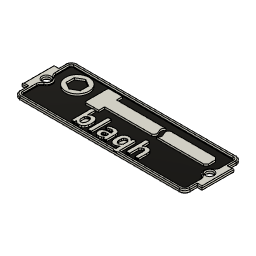
gridfinity_label_parametric_legacy (Autodesk Fusion 360 design; units mm, degrees)
Autodesk Fusion 360 part; units mm, degrees
sketch "Sketch1" plane through (0, 0, 35.65) normal (0, 0, 1) x (-1, 0, 0)
  line L0 (-2.15, 2.65) -> (-18.9, 2.65)
  line L1 (-0.25, -3.35) -> (-0.25, -0.5)
  line L2 (-1.25, -0.5) -> (-1.25, 1.5)
  arc A0 (-1.25, 1.5) -> (-2.15, 2.4) centre (-2.15, 1.5) ccw
  line L3 (-2.15, 2.4) -> (-18.9, 2.4)
  line L4 (-1.25, -0.5) -> (-0.25, -0.5)
  line L5 (0, -3.35) -> (0, 0)
  line L6 (0, 0) -> (-1, 0)
  line L7 (-1, 0) -> (-1, 1.5)
  arc A1 (-1, 1.5) -> (-2.15, 2.65) centre (-2.15, 1.5) ccw
  line L8 (-18.9, -3.35) -> (-18.9, 2.65)
  line L9 (0, -3.35) -> (-18.9, -3.35)
  line L10 (0, 0) -> (-24, 0) construction
  line L11 (0, -3.35) -> (0, -6.7)
  line L12 (-1, -6.7) -> (-1, -8.2)
  line L13 (0, -3.35) -> (-18.9, -3.35)
  line L14 (-1.25, -6.2) -> (-0.25, -6.2)
  arc A2 (-2.15, -9.35) -> (-1, -8.2) centre (-2.15, -8.2) ccw
  line L15 (-2.15, -9.35) -> (-18.9, -9.35)
  line L16 (-1.25, -6.2) -> (-1.25, -8.2)
  line L17 (0, -6.7) -> (-1, -6.7)
  arc A3 (-2.15, -9.1) -> (-1.25, -8.2) centre (-2.15, -8.2) ccw
  line L18 (-0.25, -3.35) -> (-0.25, -6.2)
  line L19 (-2.15, -9.1) -> (-18.9, -9.1)
  line L20 (-18.9, -3.35) -> (-18.9, -9.35)
  line L21 (-36.55, -6.2) -> (-37.55, -6.2)
  line L22 (-37.8, -6.7) -> (-36.8, -6.7)
  line L23 (-35.65, -9.35) -> (-18.9, -9.35)
  line L24 (-37.8, -3.35) -> (-18.9, -3.35)
  line L25 (-36.8, 0) -> (-36.8, 1.5)
  line L26 (-35.65, 2.4) -> (-18.9, 2.4)
  line L27 (-36.55, -0.5) -> (-37.55, -0.5)
  line L28 (-35.65, 2.65) -> (-18.9, 2.65)
  arc A4 (-35.65, 2.4) -> (-36.55, 1.5) centre (-35.65, 1.5) ccw
  line L29 (-37.55, -3.35) -> (-37.55, -6.2)
  line L30 (-37.55, -3.35) -> (-37.55, -0.5)
  line L31 (-37.8, -3.35) -> (-18.9, -3.35)
  line L32 (-36.55, -6.2) -> (-36.55, -8.2)
  arc A5 (-36.55, -8.2) -> (-35.65, -9.1) centre (-35.65, -8.2) ccw
  line L33 (-37.8, -3.35) -> (-37.8, 0)
  line L34 (-18.9, -3.35) -> (-18.9, 2.65)
  line L35 (-37.8, 0) -> (-36.8, 0)
  arc A6 (-35.65, 2.65) -> (-36.8, 1.5) centre (-35.65, 1.5) ccw
  arc A7 (-36.8, -8.2) -> (-35.65, -9.35) centre (-35.65, -8.2) ccw
  line L36 (-36.55, -0.5) -> (-36.55, 1.5)
  line L37 (-35.65, -9.1) -> (-18.9, -9.1)
  line L38 (-36.8, -6.7) -> (-36.8, -8.2)
  line L39 (-18.9, -3.35) -> (-18.9, -9.35)
  line L40 (-37.8, -3.35) -> (-37.8, -6.7)
  point P0 (0, -6.7)
  point P1 (0, -6.7)
  point P2 (-37.8, -6.7)
  point P3 (-37.8, -6.7)
  point P4 (-37.8, 0)
  point P5 (-37.8, 0)
  dimension "d562" = 0.25
  dimension "d566" = 0.5
  dimension "d4" = 18.9
  dimension "d5" = 3.35
  dimension "d6" = 1
  dimension "d7" = 1
  dimension "d8" = 1.15
  dimension "d9" = 0.9
  dimension "d10" = 2
  dimension "d11" = 1.5
  dimension "d12" = 0.9
  dimension "d13" = 1.15
  constraint coincident L1 L4.end
  constraint perpendicular L1 L4
  constraint tangent L2 A0
  constraint tangent A0 L3
  constraint coincident A0.centre A1.centre
  constraint coincident L5.end L6.start
  constraint coincident L8 L3.end
  constraint coincident L9 L1.start
  constraint parallel L0 L3
  constraint perpendicular L6 L7
  constraint perpendicular L5 L9
  constraint parallel L9 L10
  constraint symmetric L5.end L9 P1
  constraint symmetric L0.start L9 A2.start
  constraint symmetric L2.end L9 L16.end
  constraint symmetric A0.end L9 A3.start
  constraint symmetric A0 L9 A3
  constraint symmetric L2.start L9 L14.start
  constraint symmetric L1.end L9 L14.end
  constraint symmetric L6.end L9 L12.start
  constraint symmetric L7.end L9 L12.end
  constraint symmetric A1 L9 A2
  constraint symmetric L5.start L9 L11.start
  constraint symmetric L8.start L9 L13.end
  constraint symmetric L0.end L9 L15.end
  constraint symmetric L3.end L9 L19.end
  constraint symmetric L9 L1.start L18.start
  constraint symmetric L9 L5.end P1
  constraint symmetric L5.end L20 P5
  constraint symmetric L0.start L20 L28.start
  constraint symmetric L2.end L20 A4.end
  constraint symmetric A0.end L20 L26.start
  constraint symmetric A0 L20 A4
  constraint symmetric L2.start L20 L27.start
  constraint symmetric L1.end L20 L27.end
  constraint symmetric L6.end L20 L25.start
  constraint symmetric L7.end L20 L25.end
  constraint symmetric A1 L20 A6
  constraint symmetric L5.start L20 L24.start
  constraint symmetric L8.start L20 L9.end
  constraint symmetric L0.end L20 L8.end
  constraint symmetric L3.end L20 L26.end
  constraint symmetric L1.start L20 L29.start
  constraint symmetric L15.end L20 L23.end
  constraint symmetric A3.start L20 A5.end
  constraint symmetric L12.end L20 A7.start
  constraint symmetric P1 L20 P3
  constraint symmetric L12.start L20 L22.end
  constraint symmetric L19.end L20 L37.end
  constraint symmetric L16.end L20 L32.end
  constraint symmetric L14.end L20 L21.end
  constraint symmetric A2.start L20 L23.start
  constraint symmetric L14.start L20 L21.start
  constraint symmetric A2 L20 A7
  constraint symmetric A3 L20 A5
  constraint perpendicular L3 L34
  measures "d562" distance of L1 L5
  measures "d566" distance of L4 L6
  measures "d4" distance of L5.start L8.start
  measures "d5" distance of L5.end L5.start
  measures "d6" distance of L5.end L6.end
  measures "d7" distance of L2.start L1.end
  measures "d8" radius of A1
  measures "d9" radius of A0
  measures "d10" distance of L2.end L2.start
  measures "d11" distance of L6.end L7.end
  measures "d12" distance of L2 A0.end
  measures "d13" horizontal distance of L0.start L7.end
extrude "Extrude1" add sketch "Sketch1" along normal blind 0.4 makes body 1
sketch "Sketch2" plane through (0, 0, 36.05) normal (0, 0, 1) x (-1, 0, 0)
  line L0 (-2.15, -8.6) -> (-35.65, -8.6)
  line L1 (-36.05, -8.2) -> (-36.05, 1.5)
  line L2 (-35.65, 1.9) -> (-2.15, 1.9)
  line L3 (-1.75, 1.5) -> (-1.75, -8.2)
  arc A0 (-2.15, -8.6) -> (-1.75, -8.2) centre (-2.15, -8.2) ccw
  arc A1 (-1.75, 1.5) -> (-2.15, 1.9) centre (-2.15, 1.5) ccw
  arc A2 (-35.65, 1.9) -> (-36.05, 1.5) centre (-35.65, 1.5) ccw
  arc A3 (-36.05, -8.2) -> (-35.65, -8.6) centre (-35.65, -8.2) ccw
  circle A4 centre (-1.75, -3.35) radius 0.75
  circle A5 centre (-36.05, -3.35) radius 0.75
  circle A6 centre (-1.75, -3.35) radius 1.25
  circle A7 centre (-36.05, -3.35) radius 1.25
  arc A8 (-2.15, -9.35) -> (-1, -8.2) centre (-2.15, -8.2) ccw
  line L4 (-1, -8.2) -> (-1, -6.7)
  line L5 (-1, -6.7) -> (0, -6.7)
  line L6 (0, -6.7) -> (0, 0)
  line L7 (0, 0) -> (-1, 0)
  line L8 (-1, 0) -> (-1, 1.5)
  arc A9 (-1, 1.5) -> (-2.15, 2.65) centre (-2.15, 1.5) ccw
  arc A10 (-35.65, 2.65) -> (-36.8, 1.5) centre (-35.65, 1.5) ccw
  line L9 (-2.15, 2.65) -> (-35.65, 2.65)
  arc A11 (-35.65, 2.65) -> (-36.8, 1.5) centre (-35.65, 1.5) ccw
  line L10 (-36.8, 1.5) -> (-36.8, 0)
  line L11 (-36.8, 0) -> (-37.8, 0)
  line L12 (-37.8, 0) -> (-37.8, -6.7)
  line L13 (-37.8, -6.7) -> (-36.8, -6.7)
  line L14 (-36.8, -6.7) -> (-36.8, -8.2)
  arc A12 (-36.8, -8.2) -> (-35.65, -9.35) centre (-35.65, -8.2) ccw
  line L15 (-35.65, -9.35) -> (-2.15, -9.35)
  point P0 (-2.15, -8.2)
  dimension "d517" = 1.5
  dimension "d518" = 2.5
  constraint horizontal L0
  constraint vertical L1
  constraint horizontal L2
  constraint vertical L3
  constraint tangent L0 A0
  constraint tangent L3 A0
  constraint tangent L3 A1
  constraint tangent L2 A1
  constraint equal A0 A1
  constraint tangent L2 A2
  constraint tangent L1 A2
  constraint equal A0 A2
  constraint tangent L1 A3
  constraint tangent L0 A3
  constraint equal A0 A3
  constraint midpoint L3 A4.centre
  constraint midpoint L1 A5.centre
  constraint concentric A4 A6
  constraint concentric A5 A7
  constraint equal A4 A5
  constraint equal A6 A7
  constraint coincident P0 A0.centre
  constraint concentric A2 A10
  measures "d517" diameter of A4
  measures "d518" diameter of A6
extrude "Extrude2" add sketch "Sketch2" along normal blind 0.4 contours L3 A4 A6 | L3 A4 A6 | L1 A5 A7 | L1 A5 A7 | L3 A4 | L3 A4 | L1 A5 | L1 A5 | A8 L4 L5 L6 L7 L8 A9 A10 L9 A11 L10 L11 L12 L13 L14 A12 L15 bodies 1
fillet "Fillet2" radius 1 4 edges at (1.75, 2.1, 36.25) (1.75, 4.6, 36.25) (36.05, 2.1, 36.25) (36.05, 4.6, 36.25) on bodies 1
extrude "Extrude4" cut sketch "Sketch2" along normal through all and the other way through all contours L3 A4 | L3 A4 | L1 A5 | L1 A5 bodies 1
fillet "Fillet1" radius 0.2 2 faces at (37.4667, 3.35, 36.45) (13.4333, 3.35, 35.65) on bodies 1
sketch "Sketch3" plane through (0, 0, 36.05) normal (0, 0, 1) x (-1, 0, 0)
  line L0 (-35.65, -8.6) -> (-2.15, -8.6)
  line L1 (-2.15, 1.9) -> (-35.65, 1.9)
  line L2 (-2.15, -8.6) -> (-35.65, -8.6) construction
  line L3 (-35.65, -8.6) -> (-35.65, 1.9) construction
  line L4 (-35.65, 1.9) -> (-2.15, 1.9) construction
  line L5 (-2.15, 1.9) -> (-2.15, -8.6) construction
  line L6 (-2.15, -3.35) -> (-35.65, -3.35) construction
  arc A0 (-35.4944, -4.4698) -> (-36.05, -5.3656) centre (-35.05, -5.3656) ccw
  line L7 (-36.05, -5.3656) -> (-36.05, -8.2)
  arc A1 (-36.05, -8.2) -> (-35.65, -8.6) centre (-35.65, -8.2) ccw
  arc A2 (-2.15, -8.6) -> (-1.75, -8.2) centre (-2.15, -8.2) ccw
  line L8 (-1.75, -8.2) -> (-1.75, -5.3656)
  arc A3 (-1.75, -5.3656) -> (-2.3056, -4.4698) centre (-2.75, -5.3656) ccw
  arc A4 (-2.3056, -2.2302) -> (-2.3056, -4.4698) centre (-1.75, -3.35) ccw
  arc A5 (-2.3056, -2.2302) -> (-1.75, -1.3344) centre (-2.75, -1.3344) ccw
  line L9 (-1.75, -1.3344) -> (-1.75, 1.5)
  arc A6 (-1.75, 1.5) -> (-2.15, 1.9) centre (-2.15, 1.5) ccw
  arc A7 (-35.65, 1.9) -> (-36.05, 1.5) centre (-35.65, 1.5) ccw
  line L10 (-36.05, 1.5) -> (-36.05, -1.3344)
  arc A8 (-36.05, -1.3344) -> (-35.4944, -2.2302) centre (-35.05, -1.3344) ccw
  arc A9 (-35.4944, -4.4698) -> (-35.4944, -2.2302) centre (-36.05, -3.35) ccw
  line L11 (-2.15, -5.6) -> (-35.65, -5.6) construction
  line L12 (-18.9, -8.6) -> (-18.9, -5.6) construction
  line L13 (-18.9, -5.6) -> (-18.9, -3.35) construction
  line L14 (-34.3, -5.6) -> (-13, -5.6)
  line L15 (-13, -5.6) -> (-13, -6.85)
  line L16 (-13, -6.85) -> (-33.8, -6.85)
  line L17 (-34.3, -6.35) -> (-34.3, -5.6)
  line L18 (-13, -5.6) -> (-10, -5.6)
  line L19 (-10, -5.6) -> (-10, -7.8)
  line L20 (-10.3, -8.1) -> (-13, -8.1)
  line L21 (-13, -8.1) -> (-13, -5.6)
  circle A10 centre (-6, -5.6) radius 2.5
  line L22 (-7.5, -6.466) -> (-6, -7.3321)
  line L23 (-6, -7.3321) -> (-4.5, -6.466)
  line L24 (-4.5, -6.466) -> (-4.5, -4.734)
  line L25 (-4.5, -4.734) -> (-6, -3.8679)
  line L26 (-6, -3.8679) -> (-7.5, -4.734)
  line L27 (-7.5, -4.734) -> (-7.5, -6.466)
  arc A11 (-10.3, -8.1) -> (-10, -7.8) centre (-10.3, -7.8) ccw
  line L28 (-2.15, 1.5) -> (-35.65, 1.5) construction
  line L29 (-35.65, 1.5) -> (-35.65, -3.35) construction
  line L30 (-35.65, -3.35) -> (-2.15, -3.35) construction
  line L31 (-2.15, -3.35) -> (-2.15, 1.5) construction
  line L32 (-33.8, -6.85) -> (-34.3, -6.35)
  line L33 (-10, -5.6) -> (-10, -3.4)
  line L34 (-13, -3.1) -> (-13, -5.6)
  line L35 (-18.9, -2.6) -> (-18.9, -5.6) construction
  line L36 (-13, -4.35) -> (-33.8, -4.35)
  line L37 (-34.3, -4.85) -> (-34.3, -5.6)
  line L38 (-13, -5.6) -> (-10, -5.6)
  line L39 (-10.3, -3.1) -> (-13, -3.1)
  line L40 (-13, -5.6) -> (-13, -4.35)
  line L41 (-34.3, -5.6) -> (-13, -5.6)
  arc A12 (-10, -3.4) -> (-10.3, -3.1) centre (-10.3, -3.4) ccw
  line L42 (-33.8, -4.35) -> (-34.3, -4.85)
  point P0 (-34.3, -6.85)
  point P1 (-10, -8.1)
  point P2 (-6, -5.6)
  point P3 (-10, -3.1)
  point P4 (-34.3, -4.35)
  dimension "d21" = 3
  dimension "d22" = 0.4
  dimension "d23" = 21.3
  dimension "d24" = 3
  dimension "d25" = 1.25
  dimension "d26" = 2.5
  dimension "d31" = 5
  dimension "d33" = 1.5
  dimension "d34" = 4
  dimension "d38" = 33.5
  dimension "d39" = 1.35
  dimension "d41" = 0.3
  dimension "d43" = 4
  dimension "d44" = 0.4
  dimension "d45" = 0.5
  dimension "d46" = 0.5
  dimension "d67" = 0.4
  text T0 "blaqh" font "Calibri" height 4 bold align centre bottom in box 33.5 x 4.85 at (-2.15, 1.5) x (-1, 0) y (0, -1) spacing 1 kerned
  constraint horizontal L2
  constraint vertical L3
  constraint horizontal L4
  constraint vertical L5
  constraint midpoint L5 L6.start
  constraint midpoint L3 L6.end
  constraint coincident L5 L11.start
  constraint coincident L3 L11.end
  constraint perpendicular L3 L11
  constraint midpoint L2 L12.start
  constraint midpoint L11 L12.end
  constraint horizontal L14
  constraint vertical L15
  constraint horizontal L16
  constraint vertical L17
  constraint coincident L11 L14.start
  constraint horizontal L18
  constraint vertical L19
  constraint horizontal L20
  constraint vertical L21
  constraint coincident L11 P2
  constraint coincident P2 A10.centre
  constraint coincident P1 L19
  constraint coincident P1 L20
  constraint tangent L19 A11
  constraint tangent L20 A11
  constraint coincident L1.start L4
  constraint coincident L5
  constraint coincident L6.end
  constraint coincident P0 L16
  constraint coincident P0 L17
  constraint symmetric L11 L12.start L35.start
  constraint symmetric L11 L12.end L13.start
  constraint symmetric L11 L14.start L17.end
  constraint symmetric L11 L14.end L15.start
  constraint symmetric L11 L15.end L36.start
  constraint symmetric L11 P0 P4
  constraint symmetric L11 L18.end L19.start
  constraint symmetric L11 P1 P3
  constraint symmetric L11 L20.end L34.start
  constraint symmetric L11 L19.end L33.end
  constraint symmetric L11 L20.start L39.start
  constraint symmetric L11 A11 A12
  constraint symmetric L11 L16.end L36.end
  constraint symmetric L11 L17.start L37.start
  measures "d21" distance of L0 L11
  measures "d22" distance of L8 L11.start
  measures "d23" distance of L15.end P0
  measures "d24" distance of P1 L20.end
  measures "d25" distance of L14 L16
  measures "d26" distance of L18.end P1
  measures "d31" diameter of A10
  measures "d33" distance of P2 L27
  measures "d34" distance of L19 P2
  measures "d38" distance of L0.end L0.start
  measures "d39" distance of L3 L17
  measures "d41" radius of A11
  measures "d44" distance of L4 L28
  measures "d45" distance of P0 L16.end
  measures "d46" distance of P0 L17.start
  measures "d67" distance of L3 L7
extrude "Extrude3" add sketch "Sketch3" sketch "Sketch3" along normal blind 0.4 contours L14 L34 L36 L37 L40 L41 L42 | L14 L15 L16 L17 L21 L32 L41 | L15 L18 L19 L20 L21 A11 L38 | L18 L33 L34 L38 L39 L40 A12 | A10 of sketch 2 text T0 bodies 1
sketch "Skizze4" plane through (0, 0, 36.45) normal (0, 0, 1) x (-1, 0, 0)
  line L0 (-12.988, -6.85) -> (-12.988, -5.6) construction
  line L1 (-12.988, -5.6) -> (-34.3, -5.6) construction
  spline S0 degree 5 poles (-23.398, -6.85) (-23.3526, -6.8257) (-23.2673, -6.7758) (-23.156, -6.6971) (-23.0412, -6.5844) (-22.9541, -6.4303) (-22.9227, -6.2632) (-22.9431, -6.0841) (-23.0069, -5.8949) (-23.099, -5.6991) (-23.201, -5.5009) (-23.2931, -5.3051) (-23.3569, -5.1159) (-23.3773, -4.9368) (-23.3459, -4.7697) (-23.2588, -4.6156) (-23.144, -4.5029) (-23.0327, -4.4242) (-22.9474, -4.3743) (-22.902, -4.35) knots 0 0 0 0 0 0 0.066667 0.133333 0.2 0.266667 0.333333 0.4 0.466667 0.533333 0.6 0.666667 0.733333 0.8 0.866667 0.933333 1 1 1 1 1 1
  spline S1 degree 5 poles (-24.398, -6.85) (-24.3526, -6.8257) (-24.2673, -6.7758) (-24.156, -6.6971) (-24.0412, -6.5844) (-23.9541, -6.4303) (-23.9227, -6.2632) (-23.9431, -6.0841) (-24.0069, -5.8949) (-24.099, -5.6991) (-24.201, -5.5009) (-24.2931, -5.3051) (-24.3569, -5.1159) (-24.3773, -4.9368) (-24.3459, -4.7697) (-24.2588, -4.6156) (-24.144, -4.5029) (-24.0327, -4.4242) (-23.9474, -4.3743) (-23.902, -4.35) knots 0 0 0 0 0 0 0.066667 0.133333 0.2 0.266667 0.333333 0.4 0.466667 0.533333 0.6 0.666667 0.733333 0.8 0.866667 0.933333 1 1 1 1 1 1
  line L2 (-23.65, -5.6) -> (-22.95, -6.1)
  line L3 (-23.65, -5.6) -> (-23.95, -6.1)
  line L4 (-24.35, -5.1) -> (-23.65, -5.6)
  line L5 (-23.35, -5.1) -> (-23.65, -5.6)
  line L6 (-12.988, -5.6) -> (-12.988, -4.35) construction
  line L7 (-10, -7.8) -> (-10, -3.4)
  arc A0 (-10, -3.4) -> (-10.3, -3.1) centre (-10.3, -3.4) ccw
  line L8 (-10.3, -3.1) -> (-13, -3.1)
  line L9 (-13, -3.1) -> (-13, -4.35)
  line L10 (-13, -4.35) -> (-33.8, -4.35)
  line L11 (-33.8, -4.35) -> (-34.3, -4.85)
  line L12 (-34.3, -4.85) -> (-34.3, -6.35)
  line L13 (-34.3, -6.35) -> (-33.8, -6.85)
  line L14 (-33.8, -6.85) -> (-13, -6.85)
  line L15 (-13, -6.85) -> (-13, -8.1)
  line L16 (-13, -8.1) -> (-10.3, -8.1)
  arc A1 (-10.3, -8.1) -> (-10, -7.8) centre (-10.3, -7.8) ccw
  line L17 (-23.398, -6.85) -> (-24.398, -6.85)
  line L18 (-22.902, -4.35) -> (-23.902, -4.35)
  point P0 (-22.95, -6.1)
  point P1 (-23.35, -5.1)
  point P2 (-29.15, -5.6164)
  point P3 (-23.95, -6.1)
  point P4 (-24.35, -5.1)
  dimension "d48" = 0.5
  dimension "d49" = 0.5
  dimension "d50" = 0.448
  dimension "d51" = 0.448
  dimension "d52" = 0.4
  dimension "d56" = -1
  dimension "d57" = 0
  dimension "d70" = 10.65
  constraint coincident P4 L4.start
  constraint coincident P0 L2.end
  constraint coincident P1 L5.start
  constraint coincident P3 L3.end
  constraint equal L2 L4
  constraint equal L3 L5
  constraint equal L0 L6
  constraint perpendicular L1 L6
  constraint coincident S0.start L14
  constraint coincident S0.end L10
  constraint coincident L0.start L14
  constraint coincident L6.end L10
  constraint parallel L1 L14
  constraint parallel L0 L6
  measures "d48" distance of L1 P0
  measures "d49" distance of L1 P1
  measures "d50" distance of S0.start P0
  measures "d51" distance of P1 S0.end
  measures "d52" horizontal distance of P0 P1
  measures "d70" distance of L2.start L12
extrude "Extrusion5" add sketch "Skizze4" along normal blind 0.4 separate body contours S0 S1 L2 L3 L14 L17 | S0 L2 L5 | S0 S1 L4 L5 L10 L18 | S1 L3 L4 makes body 2
move_body "Verschieben1" bodies 2 to x (1, 0, 0) y (0, 1, 0) z (0, 0, 1) at (0, 0, -0.4)
combine "Kombinieren1" operation cut target body 1 tool bodies 2
equation "d525 = 0.0 °"
equation "d4 = ( 37.8 / 2 ) * 1 mm + ( ( Box_width - 1 ) * 42 / 2 ) * 1 mm"
equation "M = 1" comment "Nominal thread diameter"
equation "Box_width = 1"
equation "d23 = drawn_bolt_length"
equation "d24 = head_length_k"
equation "d25 = ( M_drawn / 2 )"
equation "d26 = head_diameter_dk / 2"
equation "bolt_length_l = 166 mm" comment "bolt length"
equation "head_length_k = 3 mm"
equation "head_diameter_dk = 5 mm"
equation "total_bolt_length = drawn_bolt_length + head_length_k"
equation "d31 = head_diameter_dk"
equation "Hex_width = 3 mm"
equation "d33 = Hex_width / 2"
equation "d34 = head_diameter_dk / 2 + distance_bolt_head_to_head_view"
equation "distance_bolt_head_to_head_view = 1.5 mm"
equation "total_pic_width = total_bolt_length + head_diameter_dk + distance_bolt_head_to_head_view"
equation "d39 = ( d38 - total_pic_width ) / 2"
equation "head_corner_R = 0.3 mm"
equation "d41 = head_corner_R"
equation "P = 0.5 mm" comment "Pitch"
equation "d46 = d45"
equation "d64 = if(Broken_bolt == 1; -0.400 mm; 0 mm)"
equation "Broken_bolt = if(drawn_bolt_length == bolt_length_l; 0; 1)" comment "1 to split bolt pic, 0 to keep it"
equation "drawn_bolt_length = ( if(head_diameter_dk + distance_bolt_head_to_head_view + head_length_k + bolt_length_l > d4 * 2 - 5 mm; d4 * 2 - 10 mm - head_diameter_dk - distance_bolt_head_to_head_view; bolt_length_l) )"
equation "M_drawn = 2.5 mm"
equation "d70 = drawn_bolt_length / 2"
equation "label_text = 0" comment "blaqh"
equation "text_height = 4 mm"
